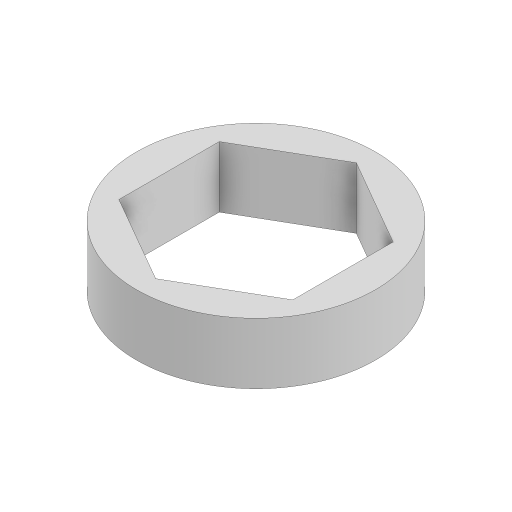
# Autodesk Inventor part: Shaft Spacers
Saved by Autodesk Inventor 2024 (Build 280153000, 153)
## iProperties
Created: 2023-01-17
Part Number: Shaft Spacers
Material: Generic
Document SubType Name: Modeling
Designer: david
Density: 1 g/cm^3
Appearance: Default
Author: david
Autodesk Inventor part; units mm, degrees
ref_plane "YZ Plane" through (0, 0, 0) normal (1, 0, 0) x (0, 1, 0)
ref_plane "XZ Plane" through (0, 0, 0) normal (0, 1, 0) x (-1, 0, 0)
ref_plane "XY Plane" through (0, 0, 0) normal (0, 0, 1) x (1, 0, 0)
sketch "Sketch1" plane through (0, 0, 0) normal (0, 1, 0) x (-1, 0, 0)
  line L0 (0, 7.5633) -> (6.55, 3.7816)
  line L1 (6.55, 3.7816) -> (6.55, -3.7816)
  line L2 (6.55, -3.7816) -> (0, -7.5633)
  line L3 (0, -7.5633) -> (-6.55, -3.7816)
  line L4 (-6.55, -3.7816) -> (-6.55, 3.7816)
  line L5 (-6.55, 3.7816) -> (0, 7.5633)
  circle A0 centre (0, 0) radius 9
  point P0 (-6.55, 0)
  point P1 (6.55, 0)
  dimension "d0" = 13.1
  dimension "d1" = 18
  constraints: 12 end point, 2 coincident, 2 midpoint, 1 centre point, 13 other
  measures "d0" distance of point (-6.55, 0) point (6.55, 0)
  measures "d1" diameter of A0
extrude "Extrusion1" add sketch "Sketch1" along normal blind 4.6
body "Solid1"
